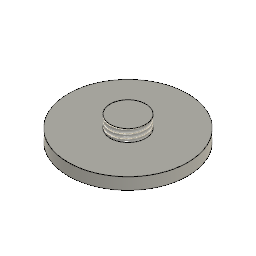
Automation dial v4 (Autodesk Fusion 360 archive; units mm, degrees)
design "Base"
Autodesk Fusion 360 part; units mm, degrees
sketch "Sketch1" plane through (0, 0, 0) normal (0, 0, 1) x (1, 0, 0)
  circle A0 centre (0, 0) radius 50
  dimension "d1" = 100
  constraint coincident A0.centre origin
  measures "d1" diameter of A0
extrude "Extrude1" add sketch "Sketch1" along normal blind 10
cylinder "CylinderPrimitive1" add diameter 30 height 10 placed x (1, 0, 0) y (0, 1, 0) z (0, 0, 1) at (0, 0, 10)
thread "Thread1" "ISO Metric profile 30.0 M30x3.5 6g" major diameter 29.7345 minor diameter 25.732 pitch 3.5 angle 60 resizes the face on face at (14.9255, -1.4935, 16.6667)

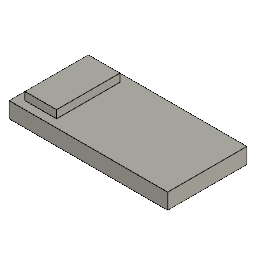
design "machine arm"
Autodesk Fusion 360 part; units mm, degrees
sketch "machine arm" plane through (0, 0, 0) normal (0, 0, 1) x (1, 0, 0)
  line L0 (-50, -25) -> (50, -25)
  line L1 (50, -25) -> (50, 25)
  line L2 (50, 25) -> (-50, 25)
  line L3 (-50, 25) -> (-50, -25)
  line L4 (-50, -25) -> (50, 25) construction
  line L5 (50, -25) -> (-50, 25) construction
  dimension "d1" = 100
  dimension "d2" = 50
  constraint horizontal L0
  constraint perpendicular L0 L1
  constraint parallel L0 L2
  constraint parallel L1 L3
  constraint coincident L4 origin
  constraint coincident L5 origin
  measures "d1" distance of L1.end L2.end
  measures "d2" distance of L0.end L1.end
extrude "Extrude1" add sketch "machine arm" along normal blind 10
sketch "socket" plane through (0, 0, 0) normal (0, 0, -1) x (1, 0, 0)
  line L0 (-50, 25) -> (-50, -25)
  line L1 (-50, -25) -> (50, -25)
  line L2 (50, -25) -> (50, 25)
  line L3 (50, 25) -> (-50, 25)
  line L4 (47.5, 10) -> (32.5, 10)
  line L5 (32.5, 10) -> (32.5, -10)
  line L6 (32.5, -10) -> (47.5, -10)
  line L7 (47.5, -10) -> (47.5, 10)
  line L8 (47.5, 10) -> (32.5, -10) construction
  line L9 (32.5, 10) -> (47.5, -10) construction
  point P0 (40, 0)
  dimension "d5" = 15
  dimension "d6" = 20
  constraint horizontal L4
  constraint perpendicular L4 L5
  constraint parallel L4 L6
  constraint parallel L5 L7
  constraint coincident L8 P0
  constraint coincident L9 P0
  measures "d5" distance of L5.end L6.end
  measures "d6" distance of L4.end L5.end
extrude "Extrude2" cut sketch "socket" against normal blind 5 contours L4 L5 L6 L7
sketch "Sketch3" plane through (0, 0, 10) normal (0, 0, 1) x (-1, 0, 0)
  line L0 (50, -25) -> (50, 25)
  line L1 (50, 25) -> (-50, 25)
  line L2 (-50, 25) -> (-50, -25)
  line L3 (-50, -25) -> (50, -25)
  line L4 (25, -20) -> (45, -20)
  line L5 (45, -20) -> (45, 20)
  line L6 (45, 20) -> (25, 20)
  line L7 (25, 20) -> (25, -20)
  point P0 (25, -20)
  constraint horizontal L4
  constraint vertical L5
  constraint horizontal L6
  constraint vertical L7
  constraint coincident P0 L4.start
extrude "Extrude3" add sketch "Sketch3" along normal blind 5 contours L4 L5 L6 L7

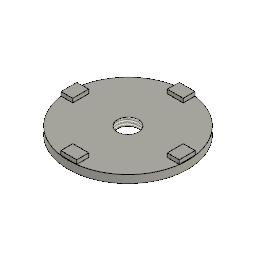
design "wheel"
Autodesk Fusion 360 part; units mm, degrees
sketch "wheel" plane through (0, 0, 0) normal (0, 0, 1) x (1, 0, 0)
  circle A0 centre (0, 0) radius 75
  dimension "d1" = 150
  constraint coincident A0.centre origin
  measures "d1" diameter of A0
extrude "Extrude1" add sketch "wheel" along normal blind 10 makes body 1
hole "Hole1" at (0, 0, 10) direction (0, 0, -1) diameter 30 depth 35 tip angle 118 bodies 1
thread "Thread1" "ISO Metric profile 30.0 M30x3.5 6H" major diameter 30.3925 minor diameter 26.491 pitch 3.5 angle 60 resizes the face on face at (0.7477, -14.9814, 6.6667) on bodies 1
ref_plane "WorkPlane1" through (0, 0, 10.25) normal (0, 0, 1) x (1, 0, 0)
sketch "connection block" plane through (0, 0, 10.25) normal (0, 0, 1) x (1, 0, 0)
  circle A0 centre (0, 0) radius 75
  line L0 (-10, 74.3303) -> (10, 74.3303)
  line L1 (10, 59.3303) -> (-10, 59.3303)
  line L2 (-10, 59.3303) -> (-10, 74.3303)
  line L3 (10, 74.3303) -> (10, 59.3303)
  line L4 (-59.3303, -10) -> (-74.3303, -10)
  line L5 (-59.3303, 10) -> (-59.3303, -10)
  line L6 (-74.3303, 10) -> (-59.3303, 10)
  line L7 (-74.3303, -10) -> (-74.3303, 10)
  line L8 (10, -59.3303) -> (10, -74.3303)
  line L9 (-10, -59.3303) -> (10, -59.3303)
  line L10 (-10, -74.3303) -> (-10, -59.3303)
  line L11 (10, -74.3303) -> (-10, -74.3303)
  line L12 (59.3303, 10) -> (74.3303, 10)
  line L13 (59.3303, -10) -> (59.3303, 10)
  line L14 (74.3303, -10) -> (59.3303, -10)
  line L15 (74.3303, 10) -> (74.3303, -10)
  point P0 (-10, 74.3303)
  point P1 (10, 74.3303)
  point P2 (10, 59.3303)
  point P3 (-9.0313, 59.3303)
  dimension "d8" = 20
  dimension "d9" = 15
  dimension "d11" = 360
  constraint coincident P0 A0
  constraint coincident A0 P1
  constraint horizontal P0 L0.end
  constraint vertical P1 P2
  constraint horizontal P2 P3
  constraint coincident P0 L0.start
  constraint coincident P1 L0.end
  constraint coincident P2 L1.start
  constraint parallel L0 L1
  constraint perpendicular L1 L2
  constraint perpendicular L1 L3
  measures "d8" distance of P0 P1
  measures "d9" distance of P1 P2
extrude "Extrude2" add sketch "connection block" along normal blind 5 separate body contours L12 L13 L14 L15 | L0 L1 L2 L3 | L8 L9 L10 L11 | L4 L5 L6 L7 makes body 2 at (69.3303, -3.3333, 10.25) makes body 3 at (3.3333, 69.3303, 10.25) makes body 4 at (-64.3303, 3.3333, 10.25) makes body 5 at (-3.3333, -69.3303, 10.25)
